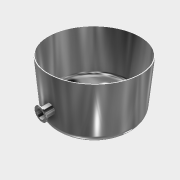
# Autodesk Inventor part: Nozzle_Template
Saved by Autodesk Inventor 2019.1 (Build 231200000, 200)
## iProperties
Created: 2009-06-25
Part Number: Nozzle_Template
Material: Steel, Mild
Document SubType Name: Modeling
Designer: Demir Ali
Mass: 9.37561e+06 g
Surface Area: 959481 cm^2
Volume: 1.19283e+06 cm^3
Density: 7.86 g/cm^3
Appearance: Chrome - Polished
Author: Demir Ali
Autodesk Inventor part; units mm, degrees
ref_plane "Work Plane4" through (-1113.6932, 1113.6932, 25) normal (0.7071068, 0.7071068, 0) x (-0.7071068, 0.7071068, 0)
ref_plane "YZ Plane" through (0, 0, 0) normal (1, 0, 0) x (0, 1, 0)
ref_plane "XZ Plane" through (0, 0, 0) normal (0, 1, 0) x (-1, 0, 0)
sketch "Sketch1" plane through (0, 0, 0) normal (0, 1, 0) x (-1, 0, 0)
  line L0 (0, 0) -> (0, 750) construction
  arc A0 (0, 750) -> (1397.2603, 1273.9726) centre (0, 2875) ccw
  arc A1 (1397.2603, 1273.9726) -> (1500, 1500) centre (1200, 1500) ccw
  line L1 (1500, 1500) -> (1500, 3000)
  line L2 (1500, 3000) -> (0, 3000)
  line L3 (0, 3000) -> (0, 750)
  dimension "d0" = 1500
  dimension "d2" = 3000
  dimension "d3" = 750
  dimension "d14" = 300
  dimension "height" = 4500
  constraints: 8 end point, 4 point on circle, 2 centre point, 2 tangent, 1 collinear, 1 parallel, 1 perpendicular, 1 point on line, 1 vertical
  measures "d0" horizontal distance of L1.start L0.start
  measures "d2" diameter of L1 L3
  measures "d3" vertical distance of L0.end L1.start
  measures "d14" radius of A1
  measures "height" diameter of L0.end L2
revolve "Revolution1" add sketch "Sketch1" angle 360 about axis through (0, 0, 3000) along (0, 0, -1)
shell "Shell1" thickness 25 removed faces 1 at (-349.4466, 349.2864, 3000)
sketch "Nozzle_SK" plane through (0, 0, 0) normal (0, 1, 0) x (-1, 0, 0)
  circle A0 centre (0, 2000) radius 161.95
  circle A1 centre (0, 2000) radius 154.85
  line L0 (0, 2000) -> (0, 0) construction
  dimension "a" = 323.9
  dimension "thk" = 7.1
  dimension "Origin_Offset" = 2000
  constraints: 2 centre point, 2 end point, 1 coincident, 1 vertical
  measures "a" diameter of A0
  measures "thk" radial gap between concentric circles of A0 A1
  measures "Origin_Offset" distance of L0.start L0.end
extrude "Nozzle_OD" add sketch "Nozzle_SK" along normal blind 1800
extrude "Nozzle_ID" cut sketch "Nozzle_SK" along normal blind 1800 contours A1
sketch "Flange_SK" plane through (0, 1800, 2000) normal (0, 1, 0) x (1, 0, 0)
  circle A0 centre (0, 0) radius 161.95
  circle A1 centre (0, 0) radius 154.85
  circle A2 centre (0, 0) radius 230
  circle A3 centre (0, 0) radius 189
  circle A4 centre (0, 0) radius 205 construction
  line L0 (0, 0) -> (0, 205) construction
  line L1 (0, 0) -> (53.0579, 198.0148) construction
  circle A5 centre (0, 0) radius 161.95 projected
  dimension "thk_z" = 7.1
  dimension "od" = 460
  dimension "k" = 410
  dimension "d1f" = 378
  dimension "angle" = 15
  dimension "az" = 323.9
  constraints: 6 coincident, 5 centre point, 4 end point, 2 point on circle, 1 vertical
  measures "thk_z" radial gap between concentric circles of A1 A0
  measures "od" diameter of A2
  measures "k" diameter of A4
  measures "d1f" diameter of A3
  measures "angle" angle of L1 L0
  measures "az" diameter of A0
extrude "Flange_OD" add sketch "Flange_SK" against normal blind 28 contours A2 | A3
chamfer "Chamfer2" distance 34 distance2 20.1 1 edges at (161.95, 1772, 2000) measured on face at (161.95, 1771.5, 2000)
extrude "Flange_Face" cut sketch "Flange_SK" against normal blind 2 contours A2
hole "Hole1" at (53.0579, 1800, 1801.9852) direction (0, -1, 0) diameter 25 depth 88 tip angle 118
pattern_circular "Circular Pattern1" count 12 over 360 about axis through (0, 0, 2000) along (0, 1, 0) of "Hole1"
extrude "Nozzle_OD_Trim" cut sketch "Nozzle_SK" along normal up to surface contours A0 | A1 round surface about axis through (0, 0, 2250) along (0, 0, -1) radius 1500 far side no
sketch3d "Sketch3"
  constraints: 4 end point, 1 perpendicular, 1 point on line
sketch3d "Sketch5"
  constraints: 32 end point, 6 parallel, 4 perpendicular, 3 equal length, 3 midpoint, 2 point on circle, 1 vertical
sketch "Sketch8" plane through (0, 0, 0) normal (1, 0, 0) x (0, 1, 0)
  arc A0 (-1326.3769, 4944.9951) -> (-1450, 4900) centre (-1380, 4900) ccw
  line L0 (-1326.3769, 4944.9951) -> (-1303.8793, 4918.1836)
  line L1 (-1450, 4865) -> (-1450, 4900)
  point P0 (0, 0)
  dimension "d98" = 70
  dimension "d101" = 35
  dimension "d102" = 1450
  dimension "d103" = 40
  dimension "d104" = 35
  dimension "d108" = 4900
  constraints: 4 end point, 2 point on circle, 2 tangent, 1 centre point, 1 vertical
  measures "d98" radius of A0
  measures "d101" distance of L0.start L0.end
  measures "d102" distance from line of L1 point (0, 0)
  measures "d103" angle of L0 L1
  measures "d104" distance of L1.start L1.end
  measures "d108" vertical distance of A0.centre point (0, 0)
ref_plane "Work Plane5" through (-1113.6932, -1113.6932, 25) normal (-0.7071068, 0.7071068, 0) x (-0.7071068, -0.7071068, 0)
ref_plane "Work Plane6" through (1113.6932, -1113.6932, 25) normal (-0.7071068, -0.7071068, 0) x (0.7071068, -0.7071068, 0)
ref_plane "Work Plane7" through (1113.6932, 1113.6932, 25) normal (0.7071068, -0.7071068, 0) x (0.7071068, 0.7071068, 0)
equation "\"d3\" = 0.25 * d2"
equation "\"d125\" = stand_off"
equation "\"thk_z\" = thk"
equation "\"az\" = a"
equation "\"d130\" = -c2 + h2 - h3"
equation "\"d131\" = n1 - a"
equation "\"d101\" = 0.5 * d98"
equation "\"d104\" = d101"
equation "\"h3\" = 16"
equation "\"n1\" = 344"
equation "\"stand_off\" = 1800"
equation "\"c2\" = 28"
equation "\"h2\" = 78"
body "Solid1"
